Autodesk Fusion 360 part; units mm, degrees
(part 11 of 11)
  arc A223 (1.92, -73.2625) -> (1.2372, -72.9797) centre (1.52, -73.2625) ccw
  line L3643 (14.02, -110.1167) -> (13.903, -109.9997)
  line L3644 (4.62, -76.6432) -> (7.1635, -74.0997)
  line L3645 (6.6572, -77.9997) -> (4.62, -77.9997)
  line L3646 (6.6572, -78.1997) -> (4.42, -78.1997)
  line L3647 (20.0587, -114.5222) -> (20.0369, -114.4741)
  line L3648 (9.92, -113.6927) -> (10.127, -113.8997)
  arc A224 (6.94, -78.6825) -> (6.6572, -77.9997) centre (6.6572, -78.3997) ccw
  line L3649 (12.7593, -113.8997) -> (16.1593, -117.2997)
  line L3650 (16.4807, -115.4997) -> (13.82, -112.839)
  line L3651 (4.42, -78.1997) -> (4.42, -76.5603)
  line L3652 (4.42, -78.1997) -> (4.42, -76.5603)
  arc A225 (1.72, -73.2625) -> (1.3786, -73.1211) centre (1.52, -73.2625) ccw
  line L3653 (19.8387, -114.5276) -> (19.8177, -114.4938)
  line L3654 (19.8387, -114.5276) -> (19.8177, -114.4938)
  point P0 (9.92, -109.9997)
  point P1 (9.92, -179.9997)
  point P2 (-0.08, -109.9997)
  point P3 (9.92, -39.9997)
  dimension "d20" = 0.2
  dimension "d21" = 0.2
  dimension "d22" = 0.2
  dimension "d23" = 0.2
  dimension "d24" = 0.2
  dimension "d25" = 0.2
  dimension "d26" = 0.2
  dimension "d27" = 0.2
  dimension "d28" = 0.2
  dimension "d29" = 0.2
  dimension "d30" = 0.2
